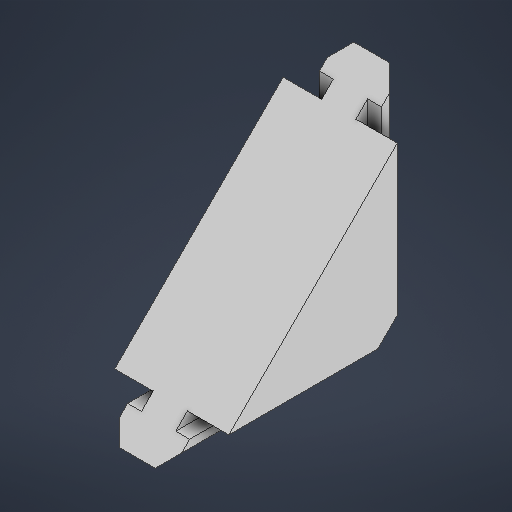
# Autodesk Inventor part: Kątownik
Saved by Autodesk Inventor 2026.1 (Build 301233020, 233B)
## iProperties
Created: 2025-12-18
Part Number: Kątownik
Material: Ogólny
Document SubType Name: Modeling
Designer: maciej
Density: 1 g/cm^3
Appearance: Domyślna
Author: maciej
Autodesk Inventor part; units mm, degrees
sketch "Szkic2" plane through (0, 0, 0) normal (0, 0, 1) x (1, 0, 0)
  circle A0 centre (0, 0) radius 2.1
  line L0 (-10, 10) -> (10, 10)
  line L1 (10, 10) -> (10, -10)
  line L2 (10, -10) -> (-10, -10)
  line L3 (-10, -10) -> (-10, 10)
  line L4 (-10, -10) -> (10, 10) construction
  line L5 (10, -10) -> (-10, 10) construction
  line L6 (-10, 8.2) -> (10, 8.2)
  line L7 (-10, -8.2) -> (10, -8.2)
  line L8 (-8.2, 10) -> (-8.2, -10)
  line L9 (10, 10) -> (30, 10)
  line L10 (30, 10) -> (30, -10)
  line L11 (30, -10) -> (10, -10)
  line L12 (10, -10) -> (10, 10)
  line L13 (-4.1857, -4.1857) -> (4.1857, -4.1857)
  line L14 (4.1857, -4.1857) -> (4.1857, 4.1857)
  line L15 (4.1857, 4.1857) -> (-4.1857, 4.1857)
  line L16 (-4.1857, 4.1857) -> (-4.1857, -4.1857)
  line L17 (-8.2, 7.1393) -> (-4.1857, 3.125)
  line L18 (-7.1393, 8.2) -> (-3.125, 4.1857)
  line L19 (-4.925, 10) -> (-3.125, 8.2)
  line L20 (4.925, 10) -> (3.125, 8.2)
  line L21 (-3.125, -8.2) -> (-4.925, -10)
  line L22 (3.125, -8.2) -> (4.925, -10)
  line L23 (-8.2, -7.1393) -> (-4.1857, -3.125)
  line L24 (-7.1393, -8.2) -> (-3.125, -4.1857)
  line L25 (3.125, -4.1857) -> (7.1393, -8.2)
  line L26 (4.1857, -3.125) -> (7.3007, -6.24)
  line L27 (4.1857, 3.125) -> (7.3007, 6.24)
  line L28 (3.125, 4.1857) -> (7.1393, 8.2)
  line L29 (-5.4993, 8.2) -> (-5.4993, 6.56)
  line L30 (5.4993, 8.2) -> (5.4993, 6.56)
  line L31 (-8.2, 5.4993) -> (-6.56, 5.4993)
  line L32 (-8.2, -5.4993) -> (-6.56, -5.4993)
  line L33 (-5.4993, -6.56) -> (-5.4993, -8.2)
  line L34 (5.4993, -6.56) -> (5.4993, -8.2)
  line L35 (-8.2, 3.125) -> (-10, 4.925)
  line L36 (-8.2, -3.125) -> (-10, -4.925)
  line L37 (7.3007, 6.24) -> (7.3007, 8.2)
  line L38 (7.3007, -6.24) -> (7.3007, -8.2)
  line L39 (15.8143, -4.1857) -> (15.8143, 4.1857)
  line L40 (24.1857, -4.1857) -> (15.8143, -4.1857)
  line L41 (23.125, -8.2) -> (24.925, -10)
  line L42 (30, -8.2) -> (10, -8.2)
  line L43 (30, 8.2) -> (10, 8.2)
  line L44 (28.2, 10) -> (28.2, -10)
  line L45 (15.8143, -3.125) -> (12.6993, -6.24)
  line L46 (27.1393, -8.2) -> (23.125, -4.1857)
  line L47 (12.6993, -6.24) -> (12.6993, -8.2)
  line L48 (16.875, -8.2) -> (15.075, -10)
  circle A1 centre (20, 0) radius 2.1
  line L49 (24.925, 10) -> (23.125, 8.2)
  line L50 (27.1393, 8.2) -> (23.125, 4.1857)
  line L51 (28.2, 7.1393) -> (24.1857, 3.125)
  line L52 (28.2, 5.4993) -> (26.56, 5.4993)
  line L53 (28.2, 3.125) -> (30, 4.925)
  line L54 (15.8143, 4.1857) -> (24.1857, 4.1857)
  line L55 (15.075, 10) -> (16.875, 8.2)
  line L56 (14.5007, 8.2) -> (14.5007, 6.56)
  line L57 (16.875, 4.1857) -> (12.8607, 8.2)
  line L58 (12.6993, 6.24) -> (12.6993, 8.2)
  line L59 (15.8143, 3.125) -> (12.6993, 6.24)
  line L60 (24.1857, 4.1857) -> (24.1857, -4.1857)
  line L61 (28.2, -7.1393) -> (24.1857, -3.125)
  line L62 (28.2, -5.4993) -> (26.56, -5.4993)
  line L63 (25.4993, -6.56) -> (25.4993, -8.2)
  line L64 (28.2, -3.125) -> (30, -4.925)
  line L65 (14.5007, -6.56) -> (14.5007, -8.2)
  line L66 (16.875, -4.1857) -> (12.8607, -8.2)
  line L67 (-13, 13) -> (33, 13)
  line L68 (33, 13) -> (33, -13)
  line L69 (33, -13) -> (-13, -13)
  line L70 (-13, -13) -> (-13, 13)
  line L71 (-10, -8.2) -> (-13, -8.2)
  line L72 (30, -8.2) -> (33, -8.2)
  line L73 (-3.125, 8.2) -> (-3.125, 10)
  line L74 (3.125, 8.2) -> (3.125, 10)
  line L75 (-8.2, 3.125) -> (-10, 3.125)
  line L76 (-8.2, -3.125) -> (-10, -3.125)
  line L77 (-3.125, -8.2) -> (-3.125, -10)
  line L78 (3.125, -8.2) -> (3.125, -10)
  line L79 (16.875, -8.2) -> (16.875, -10)
  line L80 (23.125, -8.2) -> (23.125, -10)
  line L81 (28.2, -3.125) -> (30, -3.125)
  line L82 (28.2, 3.125) -> (30, 3.125)
  line L83 (23.125, 8.2) -> (23.125, 10)
  line L84 (16.875, 8.2) -> (16.875, 10)
  line L85 (-10, 10) -> (-10, 13)
  line L86 (10, 10) -> (10, 13)
  line L87 (-5.2993, 8.2) -> (-5.2993, 6.56)
  line L88 (-6.9979, 8.3414) -> (-2.9836, 4.3271)
  line L89 (-4.3857, 4.3857) -> (4.3857, 4.3857)
  line L90 (4.3857, 4.3857) -> (4.3857, -4.3857)
  line L91 (4.3857, -4.3857) -> (-4.3857, -4.3857)
  line L92 (-4.3857, -4.3857) -> (-4.3857, 4.3857)
  line L93 (2.9836, 4.3271) -> (6.9979, 8.3414)
  line L94 (5.2993, 8.2) -> (5.2993, 6.56)
  line L95 (-10, 8) -> (10, 8)
  line L96 (10, 8) -> (30, 8)
  line L97 (2.925, 10) -> (2.925, 7.7172)
  line L98 (2.925, 7.7172) -> (5.0664, 9.8586)
  line L99 (-2.925, 10) -> (-2.925, 7.7172)
  line L100 (-2.925, 7.7172) -> (-5.0664, 9.8586)
  point P0 (0, 0)
  point P1 (0, -8.2)
  point P2 (0, 0)
  point P3 (-2.925, 8)
  point P4 (-5.2993, 8)
  point P5 (-5.2993, 6.6428)
  point P6 (-3.0422, 4.3857)
  point P7 (3.0422, 4.3857)
  point P8 (5.2993, 6.6428)
  point P9 (5.2993, 8)
  point P10 (2.925, 8)
  dimension "d2" = 4.2
  dimension "d3" = 20
  dimension "d4" = 1.8
  dimension "d5" = 20
  dimension "d6" = 20
  dimension "d7" = 1.8
  dimension "d8" = 1.8
  dimension "d9" = 1.5
  dimension "d10" = 0.75
  dimension "d11" = 135
  dimension "d12" = 6.25
  dimension "d13" = 3.125
  dimension "d14" = 1.5
  dimension "d15" = 1.5
  dimension "d16" = 1.5
  dimension "d17" = 0.75
  dimension "d18" = 0.75
  dimension "d19" = 0.75
  dimension "d20" = 1.64
  dimension "d21" = 1.64
  dimension "d22" = 1.64
  dimension "d23" = 1.64
  dimension "d24" = 1.64
  dimension "d25" = 1.64
  dimension "d26" = 45
  dimension "d27" = 1.96
  dimension "d28" = 1.96
  dimension "d29" = 3
  dimension "d30" = 3
  dimension "d31" = 3
  dimension "d32" = 3
  dimension "d49" = 0.2
  dimension "d50" = 0.2
  dimension "d51" = 0.2
  dimension "d52" = 0.2
  dimension "d53" = 0.2
  dimension "d54" = 0.2
  dimension "d55" = 0.2
  dimension "d56" = 0.2
  constraints: 196 end point, 80 point on line, 49 symmetric about line, 25 perpendicular, 19 parallel, 8 vertical, 5 horizontal, 3 coincident, 3 midpoint, 3 vertical alignment, 2 centre point, 2 horizontal alignment, 38 other
  measures "d2" diameter of A0
  measures "d3" distance of L0.start L1.start
  measures "d4" distance between parallel lines of L3 L8
  measures "d5" distance of L10.start L11.start
  measures "d6" distance between parallel lines of L10 L1
  measures "d9" distance between parallel lines of L18 L17
  measures "d10" distance between parallel lines of L18 L5
  measures "d11" angle of L0 L19
  measures "d12" distance of L22.start L21.start
  measures "d13" distance of L21.start point (0, -8.2)
  measures "d14" distance between parallel lines of L27 L28
  measures "d15" distance between parallel lines of L26 L25
  measures "d16" distance between parallel lines of L23 L24
  measures "d17" distance between parallel lines of L24 L4
  measures "d18" distance between parallel lines of L5 L26
  measures "d19" distance between parallel lines of L28 L4
  measures "d20" distance of L29.start L29.end
  measures "d21" distance of L31.start L31.end
  measures "d22" distance of L33.start L33.end
  measures "d23" distance of L32.start L32.end
  measures "d24" distance of L34.start L34.end
  measures "d25" distance of L30.start L30.end
  measures "d26" angle of L8 L35
  measures "d27" distance of L37.start L37.end
  measures "d28" distance of L26.end L38.end
  measures "d29" distance between parallel lines of L67 L0
  measures "d30" distance between parallel lines of L69 L2
  measures "d31" distance between parallel lines of L70 L3
  measures "d32" distance between parallel lines of L68 L10
  measures "d49" distance between parallel lines of L29 L87
  measures "d50" distance between parallel lines of L18 L88
  measures "d51" distance between parallel lines of L15 L89
  measures "d52" distance between parallel lines of L28 L93
  measures "d53" distance between parallel lines of L30 L94
  measures "d55" distance between parallel lines of L74 L97
  measures "d56" distance between parallel lines of L73 L99
extrude "Wyciągnięcie proste2" add sketch "Szkic2" against normal blind 40 contours L85 L67 L86 L0 | L0 L97 L6 L99 | L6 L97 L95 L99 | L100 L99 L95 L97 L98 L94 L93 L89 L88 L87 | L95 L99 L100 | L95 L98 L97
ref_plane "Płaszczyzna konstrukcyjna2" through (-4.3857, 4.3857, -40) normal (0, -0.7071, 0.7071) x (-1, 0, 0)
split "Podział1" plane through (-4.3857, 4.3857, -40) removes the side toward (0, 0.7071, -0.7071)
mirror "Odbij1" about plane through (-4.3857, 4.3857, -40) normal (0, -0.7071, 0.7071)
fillet "Zaokrąglenie1" radius 2 2 edges at (6.4625, 10, -34.3857) (-6.4625, 10, -34.3857)
sketch "Szkic7" plane through (-10, 12, -34.3857) normal (-1, 0, 0) x (0, 0, 1)
  line L0 (34.3857, -2) -> (2, -2) projected
  line L1 (34.3857, 1) -> (34.3857, -2) projected
  line L2 (34.3857, 1) -> (3, 1) projected
  arc A0 (0, 0) -> (2, -2) centre (2, 0) ccw projected
  line L3 (3, 32.3857) -> (3, 1) projected
  line L4 (3, 32.3857) -> (0, 32.3857) projected
  line L5 (0, 32.3857) -> (0, 0) projected
  point P0 (34.3857, -12)
extrude "Wyciągnięcie proste5" cut sketch "Szkic7" against normal blind 0.5
ref_plane "Płaszczyzna konstrukcyjna6" through (-4.3857, 44.3857, -40) normal (0, -0.7071, -0.7071) x (1, 0, 0)
split "Podział3" plane through (-4.3857, 44.3857, -40) removes the side toward (0, 0.7071, 0.7071)
sketch "Szkic8" plane through (10, 12, -34.3857) normal (1, 0, 0) x (0, 0, -1)
  line L0 (-25.7713, 1) -> (-28.7713, -2) projected
  line L1 (-28.7713, -2) -> (-2, -2) projected
  arc A0 (-2, -2) -> (0, 0) centre (-2, 0) ccw projected
  line L2 (0, 26.7713) -> (0, 0) projected
  line L3 (0, 26.7713) -> (-3, 23.7713) projected
  line L4 (-3, 23.7713) -> (-3, 1) projected
  line L5 (-25.7713, 1) -> (-3, 1) projected
  line L6 (-3, 23.7713) -> (-3, 1) projected
  line L7 (-25.7713, 1) -> (-3, 23.7713)
  point P0 (-34.3857, -12)
  constraints: 2 end point
extrude "Wyciągnięcie proste6" add sketch "Szkic8" against normal up to surface (19.5 mm away) contours L7 L4 L5
fillet "Zaokrąglenie3" radius 2 1 edges at (0, 4.3857, -40)
ref_plane "Work Plane7" through (-3.0422, 31.6577, -52.7279) normal (0, 0.7071, 0.7071) x (1, 0, 0)
split "Split4" plane through (-3.0422, 31.6577, -52.7279) removes the side toward (0, -0.7071, -0.7071)
